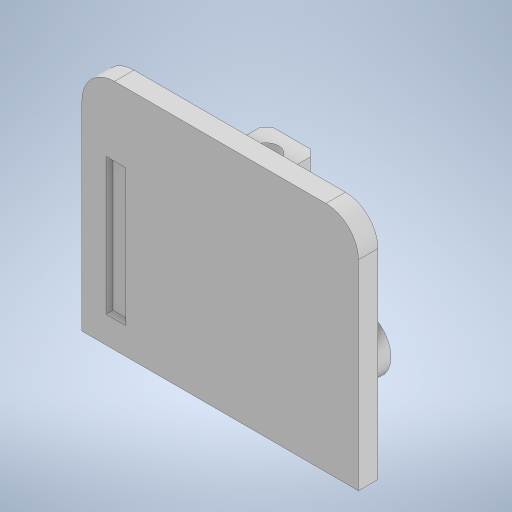
# Autodesk Inventor part: 버튼 스위치 상단
Saved by Autodesk Inventor 2023 (Build 270158000, 158)
## iProperties
Created: 2022-08-17
Part Number: 버튼 스위치 상단
Material: 일반
Document SubType Name: Modeling
Designer: user
Density: 1 g/cm^3
Appearance: 기본값
Author: user
Autodesk Inventor part; units mm, degrees
ref_plane "YZ Plane" through (0, 0, 0) normal (1, 0, 0) x (0, 1, 0)
ref_plane "XZ Plane" through (0, 0, 0) normal (0, 1, 0) x (-1, 0, 0)
sketch "스케치1" plane through (0, 0, 0) normal (0, 0, 1) x (1, 0, 0)
  line L0 (-21.25, 18.125) -> (21.25, 18.125)
  line L1 (21.25, 18.125) -> (21.25, -18.125)
  line L2 (21.25, -18.125) -> (-21.25, -18.125)
  line L3 (-21.25, -18.125) -> (-21.25, 18.125)
  line L4 (-21.25, 18.125) -> (21.25, -18.125) construction
  line L5 (21.25, 18.125) -> (-21.25, -18.125) construction
  point P0 (0, 0)
  dimension "d0" = 42.5
  dimension "d1" = 36.25
  constraints: 12 end point, 2 midpoint, 2 parallel, 1 horizontal, 1 perpendicular
  measures "d0" distance of L1.end L2.end
  measures "d1" distance of L0.end L1.end
extrude "돌출1" add sketch "스케치1" along normal blind 3
fillet "모깎기1" radius 5 2 edges at (21.25, 18.125, 1.5) (-21.25, 18.125, 1.5)
ref_plane "작업 평면1" through (-21.25, -9.325, 0) normal (0, -1, 0) x (1, 0, 0)
sketch "스케치2" plane through (-21.25, -9.325, 0) normal (0, -1, 0) x (1, 0, 0)
  line L0 (21.25, 0) -> (21.25, -4)
  circle A0 centre (21.25, -4) radius 2
  circle A1 centre (21.25, -4) radius 4
  line L1 (21.25, 0) -> (26.25, 0)
  line L2 (0, 0) -> (42.5, 0) construction
  line L3 (26.25, 0) -> (25.1524, -4.878)
  line L4 (21.25, 0) -> (16.25, 0)
  line L5 (16.25, 0) -> (17.4292, -5.184)
  dimension "d6" = 4
  dimension "d7" = 4
  dimension "d8" = 8
  dimension "d9" = 10
  constraints: 10 end point, 2 centre point, 2 coincident, 2 point on circle, 1 point on line, 1 symmetric about line, 1 tangent, 1 vertical
  measures "d6" diameter of A0
  measures "d7" distance of L0.start L0.end
  measures "d8" diameter of A1
  measures "d9" distance of L4.end L1.end
extrude "돌출2" add sketch "스케치2" along normal blind 2 contours L1 L3 A1 | A1 L5 | A1 L5 L4 picked at (20.9261, -0.7066)
pattern_linear "직사각형 패턴1" count 2 spacing 22.5 along (0, 1, 0) of "돌출2"
sketch "스케치3" plane through (0, 0, 0) normal (0, 0, -1) x (-1, 0, 0)
  circle A0 centre (16.825, -2.325) radius 4.425
  line L0 (21.25, -18.125) -> (-21.25, -18.125) projected
  line L1 (0, 0) -> (0, 4.3779)
  circle A1 centre (-16.825, -2.325) radius 4.425
  line L2 (21.25, 13.125) -> (21.25, -18.125) projected
  line L3 (-19.075, -0.075) -> (-14.575, -0.075)
  line L4 (-14.575, -0.075) -> (-14.575, -4.575)
  line L5 (-14.575, -4.575) -> (-19.075, -4.575)
  line L6 (-19.075, -4.575) -> (-19.075, -0.075)
  line L7 (-19.075, -0.075) -> (-14.575, -4.575) construction
  line L8 (-14.575, -0.075) -> (-19.075, -4.575) construction
  line L9 (14.575, -4.575) -> (19.075, -4.575)
  line L10 (19.075, -4.575) -> (19.075, -0.075)
  line L11 (19.075, -0.075) -> (14.575, -0.075)
  line L12 (14.575, -0.075) -> (14.575, -4.575)
  line L13 (14.575, -4.575) -> (19.075, -0.075) construction
  line L14 (19.075, -4.575) -> (14.575, -0.075) construction
  dimension "d16" = 15.8
  dimension "d17" = 33.65
  dimension "d18" = 4.5
  dimension "d19" = 4.5
  dimension "d20" = 4.5
  dimension "d21" = 4.5
  constraints: 26 end point, 4 midpoint, 4 parallel, 2 centre point, 2 horizontal, 2 perpendicular, 1 symmetric about line, 1 tangent, 1 vertical, 1 other
  measures "d16" distance from line of L0 A0.centre
  measures "d17" distance of A0.centre A1.centre
  measures "d18" distance of L4.end L5.end
  measures "d19" distance of L3.end L4.end
  measures "d20" distance of L11.end L10.end
  measures "d21" distance of L10.end L9.end
extrude "돌출3" add sketch "스케치3" along normal blind 2
sketch "스케치4" plane through (0, 0, 3) normal (0, 0, 1) x (1, 0, 0)
  line L0 (-21.25, -18.125) -> (21.25, -18.125) projected
  line L1 (21.25, -18.125) -> (21.25, 13.125) projected
  line L2 (-21.25, 13.125) -> (-21.25, -18.125) projected
  line L3 (-21.25, -17.625) -> (21.25, -17.625)
  point P0 (0, 0)
  dimension "d24" = 0.5
  constraints: 2 end point, 2 point on line, 1 perpendicular
  measures "d24" distance between parallel lines of L0 L3
extrude "돌출4" cut sketch "스케치4" against normal blind 3
sketch "스케치5" plane through (0, 0, 3) normal (0, 0, 1) x (1, 0, 0)
  line L0 (-17, 7) -> (-15, 7)
  line L1 (-15, 7) -> (-15, -13)
  line L2 (-15, -13) -> (-17, -13)
  line L3 (-17, -13) -> (-17, 7)
  line L4 (-17, 7) -> (-15, -13) construction
  line L5 (-15, 7) -> (-17, -13) construction
  point P0 (0, 0)
  point P1 (-16, -3)
  dimension "d27" = 2
  dimension "d28" = 20
  dimension "d32" = 3
  dimension "d37" = 16
  constraints: 12 end point, 2 midpoint, 2 parallel, 1 horizontal, 1 perpendicular
  measures "d27" distance of L0.start L0.end
  measures "d28" distance of L0.end L1.end
  measures "d32" vertical distance of point (0, 0) point (-16, -3)
  measures "d37" horizontal distance of point (-16, -3) point (0, 0)
extrude "돌출5" cut sketch "스케치5" against normal blind 0.5
chamfer "모따기1" distance 0.5 angle 45 4 edges at (-17, -3, 3) (-16, 7, 3) (-15, -3, 3) (-16, -13, 3)
sketch "스케치6" plane through (0, 0, 0) normal (0, 0, -1) x (-1, 0, 0)
  line L0 (14.575, -4.575) -> (19.075, -4.575) projected
  line L1 (19.075, -4.575) -> (19.075, -0.075) projected
  line L2 (19.075, -0.075) -> (14.575, -0.075) projected
  line L3 (14.575, -0.075) -> (14.575, -4.575) projected
  line L4 (-19.075, -0.075) -> (-19.075, -4.575) projected
  line L5 (-19.075, -4.575) -> (-14.575, -4.575) projected
  line L6 (-14.575, -4.575) -> (-14.575, -0.075) projected
  line L7 (-14.575, -0.075) -> (-19.075, -0.075) projected
  point P0 (0, 0)
extrude "돌출6" add sketch "스케치6" along normal blind 0.3
sketch "스케치7" plane through (-5, 11.175, 0) normal (0, -1, 0) x (1, 0, 0)
  arc A0 (1.1792, -5.184) -> (8.9024, -4.878) centre (5, -4) ccw projected
  line L0 (8.9024, -4.878) -> (1.1096, -4.878)
  line L1 (1.1096, -4.878) -> (1.1096, -8)
  line L2 (1.1096, -8) -> (8.9024, -8)
  line L3 (8.9024, -8) -> (8.9024, -4.878)
  line L4 (0, 0) -> (1.1792, -5.184) projected
  point P0 (5, 0)
  point P1 (5, -8)
  constraints: 8 end point, 2 parallel, 1 horizontal, 1 perpendicular, 1 point on line, 1 tangent
extrude "돌출7" add sketch "스케치7" against normal blind 2 contours A0 L2 L1 L4 | A0 L3 L2
pattern_linear "직사각형 패턴2" count 2 spacing 22.5 along (0, -1, 0) of "돌출7"
chamfer "모따기2" distance 1 angle 45 4 edges at (3.9024, 12.175, -8) (-3.8904, 12.175, -8) (3.9024, -10.325, -8) (-3.8904, -10.325, -8)
